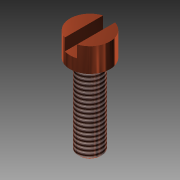
# Autodesk Inventor part: 分离前导形片固定螺丝
Saved by Autodesk Inventor 2015 (Build 190159000, 159)
## iProperties
Created: 2017-05-19
Part Number: 分离前导形片固定螺丝
Material: 常规
Document SubType Name: Modeling
Designer: Administrator
Density: 1 g/cm^3
Appearance: 铜 - 抛光
Author: Administrator
Autodesk Inventor part; units mm, degrees
ref_plane "YZ Plane" through (0, 0, 0) normal (1, 0, 0) x (0, 1, 0)
ref_plane "XZ Plane" through (0, 0, 0) normal (0, 1, 0) x (-1, 0, 0)
ref_plane "XY Plane" through (0, 0, 0) normal (0, 0, 1) x (1, 0, 0)
sketch "草图1" plane through (0, 0, 0) normal (0, 0, 1) x (1, 0, 0)
  circle A0 centre (0, 0) radius 2.5
  dimension "d0" = 5
  constraints: 1 centre point, 1 coincident
  measures "d0" diameter of A0
extrude "拉伸1" add sketch "草图1" along normal blind 3
sketch "草图2" plane through (0, 0, 3) normal (0, 0, 1) x (1, 0, 0)
  line L0 (-0.75, 2.5) -> (0.75, 2.5)
  line L1 (0.75, 2.5) -> (0.75, -2.5)
  line L2 (0.75, -2.5) -> (-0.75, -2.5)
  line L3 (-0.75, -2.5) -> (-0.75, 2.5)
  circle A0 centre (0, 0) radius 2.5 projected
  point P0 (0, 2.5)
  dimension "d3" = 1.5
  constraints: 8 end point, 3 horizontal, 2 parallel, 1 midpoint, 1 perpendicular, 1 vertical alignment, 1 other
  measures "d3" distance between parallel lines of L1 L3
extrude "拉伸2" cut sketch "草图2" against normal blind 1.5 contours L0 A0 L3 | L0 L1 A0 | A0 L1 L3 | A0 L2 L3 | L1 L2 A0
sketch "草图3" plane through (0, 0, 0) normal (0, 0, -1) x (-1, 0, 0)
  circle A0 centre (0, 0) radius 1.5
  dimension "d6" = 3
  constraints: 1 centre point, 1 coincident
  measures "d6" diameter of A0
extrude "拉伸3" add sketch "草图3" along normal blind 10
thread "螺纹1" size "M3x0.5" class "6g" standard "ANSI Metric M Profile" full length
chamfer "倒角1" distance 0.2 angle 45 1 edges at (1.5, 0, -10)
